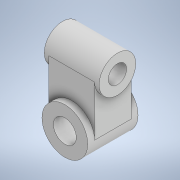
# Autodesk Inventor part: TubeSpacer
Saved by Autodesk Inventor 2022.2 (Build 262287030, 287C)
## iProperties
Created: 2023-04-24
Part Number: TubeSpacer
Material: Generic
Document SubType Name: Modeling
Designer: jak27277
Density: 1 g/cm^3
Appearance: Default
Author: jak27277
Autodesk Inventor part; units mm, degrees
ref_plane "YZ Plane" through (0, 0, 0) normal (1, 0, 0) x (0, 1, 0)
ref_plane "XZ Plane" through (0, 0, 0) normal (0, 1, 0) x (-1, 0, 0)
ref_plane "XY Plane" through (0, 0, 0) normal (0, 0, 1) x (1, 0, 0)
sketch "Sketch1" plane through (0, 0, 0) normal (0, 0, 1) x (1, 0, 0)
  circle A0 centre (0, 0) radius 31.75
  circle A1 centre (0, 0) radius 15.875
  dimension "d0" = 63.5
  dimension "d1" = 31.75
  constraints: 2 centre point, 2 coincident
  measures "d0" diameter of A0
  measures "d1" diameter of A1
extrude "Extrusion1" add sketch "Sketch1" along normal mid plane 69.85
sketch "Sketch2" plane through (0, 0, 0) normal (1, 0, 0) x (0, 1, 0)
  line L0 (0, 0) -> (69.85, 0) construction
  circle A0 centre (69.85, 0) radius 25.4
  circle A1 centre (69.85, 0) radius 12.7
  dimension "d4" = 69.85
  dimension "d5" = 50.8
  dimension "d6" = 25.4
  constraints: 2 centre point, 2 coincident, 2 end point, 1 horizontal
  measures "d4" distance of L0.start L0.end
  measures "d5" diameter of A0
  measures "d6" diameter of A1
extrude "Extrusion2" add sketch "Sketch2" along normal mid plane 76.2
sketch "Sketch3" plane through (0, 0, 0) normal (0, 1, 0) x (-1, 0, 0)
  line L0 (-31.75, -34.925) -> (31.75, -34.925) projected
  line L1 (31.75, 34.925) -> (-31.75, 34.925) projected
  line L2 (-31.75, -34.925) -> (-31.75, 34.925) projected
  line L3 (31.75, -34.925) -> (31.75, 34.925) projected
  line L4 (38.1, -25.4) -> (38.1, 25.4) projected
  line L5 (-38.1, 25.4) -> (-38.1, -25.4) projected
  line L6 (38.1, 25.4) -> (-38.1, 25.4) projected
  line L7 (38.1, -25.4) -> (-38.1, -25.4) projected
  line L8 (31.75, 25.4) -> (-31.75, 25.4)
  line L9 (-31.75, -25.4) -> (-31.75, 25.4)
  line L10 (-31.75, -25.4) -> (31.75, -25.4)
  line L11 (31.75, 25.4) -> (31.75, -25.4)
  point P0 (0, 0)
  constraints: 8 end point, 8 point on line, 2 collinear
extrude "Extrusion3" add sketch "Sketch3" along normal up to surface contours L2 L6 L3 L7
sketch "Sketch4" plane through (0, 0, 34.925) normal (0, 0, 1) x (1, 0, 0)
  circle A0 centre (0, 0) radius 15.875
  constraints: 1 centre point, 1 coincident
extrude "Extrusion4" cut sketch "Sketch4" against normal through all
body "Solid1"
